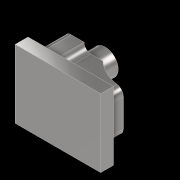
# Autodesk Inventor part: P2
Saved by Autodesk Inventor 2020 (Build 240168000, 168)
## iProperties
Created: 2021-01-27
Part Number: P2
Material: Generic
Document SubType Name: Modeling
Designer: Pedro Barriviera
Density: 1 g/cm^3
Appearance: Galvanized
Author: Pedro Barriviera
Autodesk Inventor part; units mm, degrees
ref_plane "YZ Plane" through (0, 0, 0) normal (1, 0, 0) x (0, 1, 0)
ref_plane "XZ Plane" through (0, 0, 0) normal (0, 1, 0) x (-1, 0, 0)
ref_plane "XY Plane" through (0, 0, 0) normal (0, 0, 1) x (1, 0, 0)
sketch "Sketch1" plane through (0, 0, 0) normal (0, 0, 1) x (1, 0, 0)
  line L0 (-50, 40) -> (50, 40)
  line L1 (50, 40) -> (50, -40)
  line L2 (50, -40) -> (-50, -40)
  line L3 (-50, -40) -> (-50, 40)
  line L4 (-50, 40) -> (50, -40) construction
  line L5 (50, 40) -> (-50, -40) construction
  line L6 (-34.5, 32.5) -> (-19.5, 32.5)
  line L7 (-19.5, -32.5) -> (-34.5, -32.5)
  line L8 (-42.5, -24.5) -> (-42.5, 24.5)
  line L9 (-42.5, 32.5) -> (-19.5, -32.5) construction
  line L10 (-19.5, 32.5) -> (-42.5, -32.5) construction
  arc A0 (-34.5, 32.5) -> (-42.5, 24.5) centre (-34.5, 24.5) ccw
  arc A1 (-42.5, -24.5) -> (-34.5, -32.5) centre (-34.5, -24.5) ccw
  line L11 (-11.5, 24.5) -> (34.5, 24.5)
  line L12 (42.5, 16.5) -> (42.5, -16.5)
  line L13 (34.5, -24.5) -> (-11.5, -24.5)
  line L14 (-19.5, 24.5) -> (42.5, -24.5) construction
  line L15 (42.5, 24.5) -> (-19.5, -24.5) construction
  arc A2 (42.5, 16.5) -> (34.5, 24.5) centre (34.5, 16.5) ccw
  arc A3 (34.5, -24.5) -> (42.5, -16.5) centre (34.5, -16.5) ccw
  arc A4 (-19.5, 32.5) -> (-11.5, 24.5) centre (-11.5, 32.5) ccw
  arc A5 (-11.5, -24.5) -> (-19.5, -32.5) centre (-11.5, -32.5) ccw
  circle A6 centre (-19.5, 0) radius 15
  line L16 (17.5, 15) -> (29.5, 15)
  line L17 (29.5, 15) -> (29.5, -15)
  line L18 (29.5, -15) -> (17.5, -15)
  line L19 (9.5, -7) -> (9.5, 7)
  line L20 (9.5, 15) -> (29.5, -15) construction
  line L21 (29.5, 15) -> (9.5, -15) construction
  arc A7 (17.5, 15) -> (9.5, 7) centre (17.5, 7) ccw
  arc A8 (9.5, -7) -> (17.5, -15) centre (17.5, -7) ccw
  point P0 (0, 0)
  point P1 (-31, 0)
  point P2 (11.5, 0)
  point P3 (19.5, 0)
  dimension "d0" = 100
  dimension "d1" = 80
  dimension "d2" = 23
  dimension "d3" = 65
  dimension "d4" = 8
  dimension "d5" = 8
  dimension "d6" = 7.5
  dimension "d7" = 62
  dimension "d8" = 49
  dimension "d9" = 7.5
  dimension "d10" = 8
  dimension "d13" = 30
  dimension "d14" = 23
  dimension "d15" = 20
  dimension "d16" = 30
  dimension "d17" = 13
  dimension "d18" = 8
  dimension "d32" = 8
  dimension "d34" = 46
  dimension "d35" = 8
  constraints: 44 end point, 16 point on circle, 14 tangent, 12 point on line, 9 centre point, 6 midpoint, 6 parallel, 4 horizontal, 3 perpendicular, 2 equal radius
  measures "d0" distance of L1.end L2.end
  measures "d1" distance of L0.end L1.end
  measures "d2" distance of L7.start L10.end
  measures "d3" distance of L6.end L7.start
  measures "d4" radius of A0
  measures "d5" radius of A1
  measures "d6" distance between parallel lines of L3 L8
  measures "d7" distance of L15.end L14.end
  measures "d8" distance of L15.start L14.end
  measures "d9" distance between parallel lines of L1 L12
  measures "d10" radius of A2
  measures "d13" diameter of A6
  measures "d14" distance from line of L8 A6.centre
  measures "d15" distance of L17.end L21.end
  measures "d16" distance of L16.end L17.end
  measures "d17" distance between parallel lines of L12 L17
  measures "d18" radius of A7
  measures "d32" radius of A4
  measures "d34" distance of L13.start L13.end
  measures "d35" radius of A5
extrude "Extrusion1" add sketch "Sketch1" along normal blind 15 contours L0 L1 L2 L3 | L6 A4 L11 A2 L12 A3 L13 A5 L7 A1 L8 A0 | A6 | L16 L17 L18 A8 L19 A7
extrude "Extrusion2" add sketch "Sketch1" against normal blind 60 contours A6
extrude "Extrusion3" add sketch "Sketch1" against normal blind 35 contours L6 A4 L11 A2 L12 A3 L13 A5 L7 A1 L8 A0
extrude "Extrusion4" add sketch "Sketch1" against normal blind 19 contours L16 L17 L18 A8 L19 A7
sketch "Sketch2" plane through (-11.5, 24.5, 0) normal (0, 1, 0) x (1, 0, 0)
  circle A0 centre (54.7979, 78.9947) radius 60
  line L0 (46, 0) -> (54, 0) projected
  line L1 (54, 0) -> (54, 19)
  line L2 (54, 0) -> (54, 35) projected
  line L3 (54, 35) -> (14, 35)
  line L4 (0, 35) -> (46, 35) projected
  point P0 (11.5, 0)
  dimension "d27" = 120
  dimension "d28" = 19
  dimension "d29" = 40
  constraints: 4 end point, 2 point on circle, 2 point on line, 1 centre point
  measures "d27" diameter of A0
  measures "d28" distance of L0.end L1.end
  measures "d29" distance of L2.end L3.end
extrude "Extrusion5" cut sketch "Sketch2" against normal blind 60 contours L3 L2 A0 picked at (26.9594, 33.1676)
body "Solid1"
